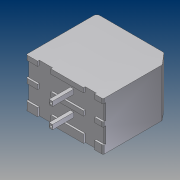
# Autodesk Inventor part: 739-302
Saved by Autodesk Inventor 2012 (Build 160160000, 160)
## iProperties
Category: PARTsolutions
Company: Team 801
Created: 2008-05-31
Part Number: 739-302
Catalog Web Link: www.team801.org
Description: 739-302 TO 739-312 - PCB TERMINAL STRIP 1 SOLDER PIN / POLE PIN SPACING 3.5 MM / 0.138 IN
Document SubType Name: Modeling
Designer: Jeffrey M
Mass: 1.27941 g
Surface Area: 8.52476 cm^2
Volume: 1.27941 cm^3
Density: 1 g/cm^3
Material: Default
NB: 739-302
NN: 739-302 TO 739-312
NT: PCB TERMINAL STRIP 1 SOLDER PIN / POLE PIN SPACING 3.5 MM / 0.138 IN
NBSYN: $BESTNR.
LINA: 739-302
BESTNR: 739-302
QUERSCHNITT1: 0.08 - 1.5
QUERSCHNITT2: 28 - 14
ABISOLIERLAENGE: 5 - 6
SPANNUNG: 250
BEMESSSTOSSSPG: 3
VERSCHMUTZGRAD: 2
STROM: 6
RM: 3.50
P: 2
HOEHE: 12.30
BREITE: 8.50
TIEFE: 13.40
ANZAHLKLEMMSTEL: 2
ANZAHLPOTENTIAL: 2
FARBE: grau
GEWICHT: 1.413
EAN: 4044918301312
BEMERKUNGEN: L = (No. of poles x Pin Spacing) + 1,5 mm
BOHRLOCHDURCHM: 1,1 +0,1 mm
RGB: 0.67,0.67,0.67,0
KT: DUMMY
PSOL_IDENT_0: {\\partserver001.servicenet\dplatte\cadenas\23d-libs\wago\pg04\serie739\0739-0302_0999-0962.prj},160
PSOL_IDENT_1: {VTYP=3D},{NB=739-302},{LINA=739-302},{NN=739-302 TO 739-312},{DATE=10.04.2007 09:24:23},{GEOMDATE=
PSOL_IDENT_2: 13.06.2006},{VERSION=},{LINEID=160},{LINESUBID=-1},{WBVAR=}  {NB=739-302},{LINA=739-302},{KT=DUMMY},
PSOL_IDENT_3: {BESTNR=739-302},{QUERSCHNITT1=0.08 - 1.5},{QUERSCHNITT2=28 - 14},{ABISOLIERLAENGE=5 - 6},{SPANNUNG=
PSOL_IDENT_4: 250},{BEMESSSTOSSSPG=3},{VERSCHMUTZGRAD=2},{STROM=6},{RM=3.50},{P=2},{HOEHE=12.30},{BREITE=8.50},{TI
PSOL_IDENT_5: EFE=13.40},{ANZAHLKLEMMSTEL=2},{ANZAHLPOTENTIAL=2},{FARBE=grau},{GEWICHT=1.413},{EAN=4044918301312},
PSOL_IDENT_6: {BEMERKUNGEN=L = (No. of poles x Pin Spacing) + 1,5 mm},{BOHRLOCHDURCHM=1,1 +0,1 mm},{RGB=0.67,0.67,
PSOL_IDENT_7: 0.67,0}
Title: 739-302
Author: Jeffrey M
Comments: PCB TERMINAL STRIP 1 SOLDER PIN / POLE PIN SPACING 3.5 MM / 0.138 IN
Autodesk Inventor part; units mm, degrees
ref_plane "YZ Plane" through (0, 0, 0) normal (1, 0, 0) x (0, 1, 0)
ref_plane "XZ Plane" through (0, 0, 0) normal (0, 1, 0) x (-1, 0, 0)
ref_plane "XY Plane" through (0, 0, 0) normal (0, 0, 1) x (1, 0, 0)
sketch "Skizze_1" plane through (0, 0, 0) normal (0, 0, 1) x (1, 0, 0)
  arc A0 (-7.7, 0.5) -> (-7.5, 0.3) centre (-7.5, 0.5) ccw
  line L0 (-7.5, 0.3) -> (5.5, 0.3)
  arc A1 (5.5, 0.3) -> (5.7, 0.5) centre (5.5, 0.5) ccw
  line L1 (5.7, 0.5) -> (5.7, 10.1162)
  arc A2 (5.7, 10.1162) -> (5.581, 10.44) centre (5.2, 10.1162) ccw
  line L2 (5.581, 10.44) -> (4.1497, 12.1238)
  arc A3 (4.1497, 12.1238) -> (3.7688, 12.3) centre (3.7688, 11.8) ccw
  line L3 (3.7688, 12.3) -> (-7.2, 12.3)
  arc A4 (-7.2, 12.3) -> (-7.7, 11.8) centre (-7.2, 11.8) ccw
  line L4 (-7.7, 11.8) -> (-7.7, 0.5)
  constraints: 10 end point, 10 point on circle, 5 centre point
extrude "Extrusion1" add sketch "Skizze_1" along normal blind 7
sketch "Skizze_2" plane through (0, 0, 7) normal (0, 0, 1) x (1, 0, 0)
  line L0 (4.2, 0) -> (5.5, 0)
  arc A0 (5.5, 0) -> (5.7, 0.2) centre (5.5, 0.2) ccw
  line L1 (5.7, 0.2) -> (5.7, 0.5)
  line L2 (5.7, 0.5) -> (4.2, 0.5)
  line L3 (4.2, 0.5) -> (4.2, 0)
  constraints: 8 end point, 2 point on circle, 1 centre point
extrude "Extrusion2" add sketch "Skizze_2" against normal blind 0.8
pattern_linear "Rectangular Pattern1" count 2 spacing 3.5 along (0, 0, -1) of "Extrusion2"
sketch "Skizze_4" plane through (0, 0, 7) normal (0, 0, 1) x (1, 0, 0)
  line L0 (-7.7, 1) -> (-7.7, 0.2)
  arc A0 (-7.7, 0.2) -> (-7.5, 0) centre (-7.5, 0.2) ccw
  line L1 (-7.5, 0) -> (-5.7, 0)
  line L2 (-5.7, 0) -> (-5.7, 1)
  line L3 (-5.7, 1) -> (-7.7, 1)
  constraints: 8 end point, 2 point on circle, 1 centre point
extrude "Extrusion3" add sketch "Skizze_4" against normal blind 0.8
pattern_linear "Rectangular Pattern2" count 2 spacing 3.5 along (0, 0, -1) of "Extrusion3"
sketch "Skizze_6" plane through (0, 0, 7) normal (0, 0, 1) x (1, 0, 0)
  line L0 (-3.4, 0) -> (2.3, 0)
  line L1 (2.3, 0) -> (2.3, 1)
  line L2 (2.3, 1) -> (-3.4, 1)
  line L3 (-3.4, 1) -> (-3.4, 0)
  constraints: 8 end point
extrude "Extrusion4" add sketch "Skizze_6" against normal blind 0.8
pattern_linear "Rectangular Pattern3" count 2 spacing 3.5 along (0, 0, -1) of "Extrusion4"
sketch "Skizze_8" plane through (0, 0, 0) normal (0, 0, 1) x (1, 0, 0)
  circle A0 centre (4.3, 1.6) radius 0.6
  constraints: 1 centre point
extrude "Extrusion5" add sketch "Skizze_8" against normal blind 1.5
sketch "Skizze_9" plane through (0, 0, 0) normal (0, 0, 1) x (1, 0, 0)
  circle A0 centre (4.3, 4.7) radius 0.6
  constraints: 1 centre point
extrude "Extrusion6" add sketch "Skizze_9" against normal blind 1.5
sketch "Skizze_10" plane through (0, 0, 0) normal (0, 0, 1) x (1, 0, 0)
  circle A0 centre (4.3, 8.3) radius 0.6
  constraints: 1 centre point
extrude "Extrusion7" add sketch "Skizze_10" against normal blind 1.5
sketch "Skizze_11" plane through (0, 0, 0) normal (0, 0, 1) x (1, 0, 0)
  circle A0 centre (-6, 1.6) radius 0.5
  constraints: 1 centre point
extrude "Extrusion8" add sketch "Skizze_11" against normal blind 1.5
sketch "Skizze_12" plane through (0, 0, 0) normal (0, 0, 1) x (1, 0, 0)
  circle A0 centre (-6, 3.4) radius 0.5
  constraints: 1 centre point
extrude "Extrusion9" add sketch "Skizze_12" against normal blind 1.5
sketch "Skizze_13" plane through (0, 0, 0) normal (0, 0, 1) x (1, 0, 0)
  circle A0 centre (-6.5, 8.9) radius 0.5
  constraints: 1 centre point
extrude "Extrusion10" add sketch "Skizze_13" against normal blind 1.5
sketch "Skizze_14" plane through (0, 0, 0) normal (0, 0, 1) x (1, 0, 0)
  circle A0 centre (-6.5, 10.8) radius 0.5
  constraints: 1 centre point
extrude "Extrusion11" add sketch "Skizze_14" against normal blind 1.5
sketch "Skizze_15" plane through (0, 0, 0) normal (0, 0, 1) x (1, 0, 0)
  arc A0 (-7.7, 0.2) -> (-7.5, 0) centre (-7.5, 0.2) ccw
  line L0 (-7.5, 0) -> (-5.7, 0)
  line L1 (-5.7, 0) -> (-5.7, 0.3)
  line L2 (-5.7, 0.3) -> (-3.4, 0.3)
  line L3 (-3.4, 0.3) -> (-3.4, 0)
  line L4 (-3.4, 0) -> (2.3, 0)
  line L5 (2.3, 0) -> (2.3, 0.3)
  line L6 (2.3, 0.3) -> (4.2, 0.3)
  line L7 (4.2, 0.3) -> (4.2, 0)
  line L8 (4.2, 0) -> (5.5, 0)
  arc A1 (5.5, 0) -> (5.7, 0.2) centre (5.5, 0.2) ccw
  line L9 (5.7, 0.2) -> (5.7, 10.1162)
  arc A2 (5.7, 10.1162) -> (5.581, 10.44) centre (5.2, 10.1162) ccw
  line L10 (5.581, 10.44) -> (4.1497, 12.1238)
  arc A3 (4.1497, 12.1238) -> (3.7688, 12.3) centre (3.7688, 11.8) ccw
  line L11 (3.7688, 12.3) -> (-7.2, 12.3)
  arc A4 (-7.2, 12.3) -> (-7.7, 11.8) centre (-7.2, 11.8) ccw
  line L12 (-7.7, 11.8) -> (-7.7, 0.2)
  constraints: 26 end point, 10 point on circle, 5 centre point
extrude "Extrusion12" add sketch "Skizze_15" against normal blind 1.4
sketch "Skizze_16" plane through (0, 0, 0) normal (0, 0, 1) x (1, 0, 0)
  line L0 (-5.8, 12.3) -> (-5.5, 12)
  line L1 (-5.5, 12) -> (-5.5, 10.8)
  line L2 (-5.5, 10.8) -> (-2.6, 10.8)
  line L3 (-2.6, 10.8) -> (-2.6, 12)
  line L4 (-2.6, 12) -> (-2.3, 12.3)
  line L5 (-2.3, 12.3) -> (-5.8, 12.3)
  constraints: 12 end point
extrude "Extrusion13" cut sketch "Skizze_16" along normal blind 3.2
pattern_linear "Rectangular Pattern4" count 2 spacing 3.5 along (0, 0, 1) of "Extrusion13"
sketch "Skizze_18" plane through (0, 0, 0) normal (1, 0, 0) x (0, 1, 0)
  line L0 (10.8, 3.2) -> (10.8, 2.9)
  line L1 (10.8, 2.9) -> (12, 2.9)
  line L2 (12, 2.9) -> (12.3, 3.2)
  line L3 (12.3, 3.2) -> (10.8, 3.2)
  constraints: 8 end point
extrude "Extrusion14" add sketch "Skizze_18" against normal blind 6
pattern_linear "Rectangular Pattern5" count 2 spacing 3.5 along (0, 0, 1) of "Extrusion14"
sketch "Skizze_20" plane through (-0.9, 0, 0) normal (1, 0, 0) x (0, 0, -1)
  line L0 (-3.2, 12.3) -> (-2.6, 10.3)
  line L1 (-2.6, 10.3) -> (-0.8, 10.3)
  line L2 (-0.8, 10.3) -> (0, 12.3)
  line L3 (0, 12.3) -> (-3.2, 12.3)
  constraints: 8 end point
extrude "Extrusion15" cut sketch "Skizze_20" along normal blind 4.1
pattern_linear "Rectangular Pattern6" count 2 spacing 3.5 along (0, 0, 1) of "Extrusion15"
sketch "Skizze_22" plane through (0, 0, 0) normal (0, 0, 1) x (1, 0, 0)
  line L0 (-0.9, 9.8) -> (3.2, 9.8)
  line L1 (3.2, 9.8) -> (3.2, 12.3)
  line L2 (3.2, 12.3) -> (2.7, 10.3)
  line L3 (2.7, 10.3) -> (-0.35, 10.3)
  line L4 (-0.35, 10.3) -> (-0.9, 12.3)
  line L5 (-0.9, 12.3) -> (-0.9, 9.8)
  constraints: 12 end point
extrude "Extrusion16" add sketch "Skizze_22" along normal blind 7
sketch "Skizze_23" plane through (-0.9, 0, 0) normal (1, 0, 0) x (0, 0, -1)
  line L0 (-1.7, 10.3) -> (-1.7, 12.3)
  line L1 (-1.7, 12.3) -> (-0.7, 12.3)
  line L2 (-0.7, 12.3) -> (-1, 10.3)
  line L3 (-1, 10.3) -> (-1.7, 10.3)
  line L4 (-1.7, 10.3) -> (-1.7, 12.3)
  constraints: 10 end point
revolve "Revolution1" cut sketch "Skizze_23" angle 360 about axis through (-0.9, 10.3, 1.7) along (0, -1, 0)
pattern_linear "Rectangular Pattern7" count 2 spacing 3.5 along (0, 0, 1) of "Revolution1"
sketch "Skizze_24" plane through (-0.9, 0, 0) normal (1, 0, 0) x (0, 0, -1)
  line L0 (-2.7, 12.3) -> (-2.4, 10.3)
  line L1 (-2.4, 10.3) -> (-1, 10.3)
  line L2 (-1, 10.3) -> (-0.7, 12.3)
  line L3 (-0.7, 12.3) -> (-2.7, 12.3)
  constraints: 8 end point
extrude "Extrusion17" cut sketch "Skizze_24" along normal blind 1
pattern_linear "Rectangular Pattern8" count 2 spacing 3.5 along (0, 0, 1) of "Extrusion17"
sketch "Skizze_27" plane through (0, 0.3, 0) normal (0, 1, 0) x (1, 0, 0)
  line L0 (-0.3, -1.35) -> (-0.3, -2.15)
  line L1 (-0.3, -2.15) -> (0.3, -2.15)
  line L2 (0.3, -2.15) -> (0.3, -1.35)
  line L3 (0.3, -1.35) -> (-0.3, -1.35)
  constraints: 8 end point
extrude "Extrusion18" add sketch "Skizze_27" against normal blind 3.7
pattern_linear "Rectangular Pattern9" count 2 spacing 3.5 along (0, 0, 1) of "Extrusion18"
sketch "Sketch20" plane through (-0.3, -3.4, 5.65) normal (0, -1, 0) x (1, 0, 0)
  line L0 (0, 0) -> (0.6, 0) construction
  line L1 (0.6, -0.8) -> (0, -0.8) construction
  line L2 (0, -3.5) -> (0.6, -3.5) construction
  line L3 (0.6, -4.3) -> (0, -4.3) construction
  line L4 (0, -3.5) -> (0.6, -4.3) construction
  line L5 (0, 0) -> (0.6, -0.8) construction
  circle A0 centre (0.3, -0.4) radius 0.25
  circle A1 centre (0.3, -3.9) radius 0.25
  point P0 (0.3, -5.65)
  dimension "d91" = 0.5
  constraints: 4 end point, 2 centre point, 2 midpoint, 1 equal radius, 1 parallel
  measures "d91" diameter of A0
extrude "Extrusion19" cut sketch "Sketch20" against normal blind 0.5
body "Solid1"
